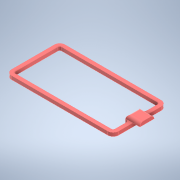
# Autodesk Inventor part: SolarpanelAdapter_bot
Saved by Autodesk Inventor 2022 (Build 260153000, 153)
## iProperties
Created: 2022-05-31
Part Number: SolarpanelAdapter_bot
Material: ABS Plastic
Document SubType Name: Modeling
Designer: Sergey
Density: 1.06 g/cm^3
Appearance: Smooth - Red
Author: Sergey
Autodesk Inventor part; units mm, degrees
ref_plane "YZ Plane" through (0, 0, 0) normal (1, 0, 0) x (0, 1, 0)
ref_plane "XZ Plane" through (0, 0, 0) normal (0, 1, 0) x (-1, 0, 0)
ref_plane "XY Plane" through (0, 0, 0) normal (0, 0, 1) x (1, 0, 0)
sketch "Sketch1" plane through (0, 0, 0) normal (0, 1, 0) x (-1, 0, 0)
  line L0 (-27, 15) -> (27, 15)
  line L1 (30, 12) -> (30, -12)
  line L2 (27, -15) -> (-27, -15)
  line L3 (-30, -12) -> (-30, 12)
  line L4 (-30, 15) -> (30, -15) construction
  line L5 (30, 15) -> (-30, -15) construction
  arc A0 (30, 12) -> (27, 15) centre (27, 12) ccw
  arc A1 (27, -15) -> (30, -12) centre (27, -12) ccw
  arc A2 (-30, -12) -> (-27, -15) centre (-27, -12) ccw
  arc A3 (-27, 15) -> (-30, 12) centre (-27, 12) ccw
  line L6 (28, -12) -> (28, 12)
  arc A4 (28, 12) -> (27, 13) centre (27, 12) ccw
  line L7 (27, 13) -> (-27, 13)
  arc A5 (-27, 13) -> (-28, 12) centre (-27, 12) ccw
  line L8 (-28, 12) -> (-28, -12)
  arc A6 (-28, -12) -> (-27, -13) centre (-27, -12) ccw
  line L9 (-27, -13) -> (27, -13)
  arc A7 (27, -13) -> (28, -12) centre (27, -12) ccw
  line L10 (-26, -4) -> (-30, -4)
  line L11 (-30, -4) -> (-30, 4)
  line L12 (-30, 4) -> (-26, 4)
  line L13 (-26, 4) -> (-26, -4)
  line L14 (-26, -4) -> (-30, 4) construction
  line L15 (-30, -4) -> (-26, 4) construction
  point P0 (0, 0)
  point P1 (-28, 0)
  point P2 (-28, 4)
  point P3 (-28, -4)
  dimension "d0" = 30
  dimension "d1" = 60
  dimension "d2" = 3
  dimension "d3" = 3
  dimension "d4" = 2
  dimension "d7" = 8
  constraints: 32 end point, 16 point on circle, 9 point on line, 8 centre point, 8 tangent, 6 parallel, 5 midpoint, 3 perpendicular, 2 equal radius, 2 horizontal, 7 other
  measures "d0" distance of L5.start L4.end
  measures "d1" distance of L4.end L5.end
  measures "d2" radius of A0
  measures "d3" radius of A1
  measures "d4" distance between parallel lines of L1 L6
  measures "d7" distance of L10.end L11.end
extrude "Extrusion1" add sketch "Sketch1" along normal blind 2 contours L0 A0 L1 A1 L2 A2 L3 L10 L8 A6 L9 A7 L6 A4 L7 A5 L12 A3 | L12 L8 L10 L3 | L12 L13 L10 L8
sketch "Sketch2" plane through (0, 2, 0) normal (0, 1, 0) x (1, 0, 0)
  line L0 (26, -4) -> (28, -4) projected
  line L1 (34, 4) -> (26, 4)
  line L2 (26, 4) -> (26, -4)
  line L3 (26, -4) -> (34, -4)
  line L4 (34, -4) -> (34, 4)
  line L5 (30, -12) -> (30, 12) projected
  line L6 (34, 4) -> (26, -4) construction
  line L7 (26, 4) -> (34, -4) construction
  point P0 (0, 0)
  point P1 (30, 0)
  constraints: 12 end point, 3 midpoint, 2 parallel, 1 horizontal, 1 perpendicular
extrude "Extrusion2" add sketch "Sketch2" along normal blind 2
fillet "Fillet1" radius 2 3 edges at (26, 4, 0) (30, 4, -4) (30, 4, 4)
fillet "Fillet2" radius 2 2 edges at (28, 1, -4) (28, 1, 4)
body "Solid1"
